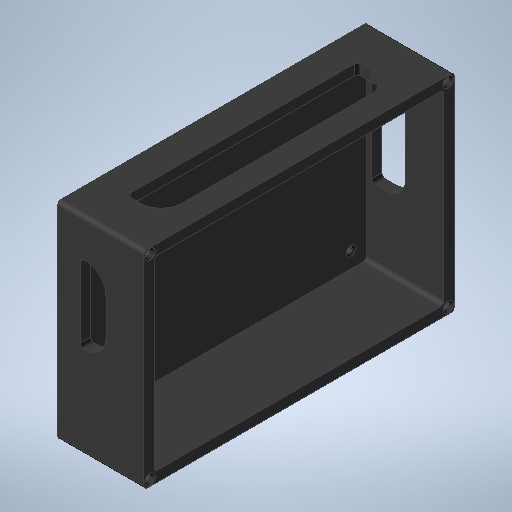
# Autodesk Inventor part: OCTOPUS_BOX
Saved by Autodesk Inventor 2025.2 (Build 292293000, 293)
## iProperties
Created: 2026-03-25
Part Number: OCTOPUS_BOX
Material: Generic
Document SubType Name: Modeling
Designer: composite
Density: 1 g/cm^3
Appearance: Default
Author: composite
Autodesk Inventor part; units mm, degrees
ref_plane "YZ Plane" through (0, 0, 0) normal (1, 0, 0) x (0, 1, 0)
ref_plane "XZ Plane" through (0, 0, 0) normal (0, 1, 0) x (-1, 0, 0)
ref_plane "XY Plane" through (0, 0, 0) normal (0, 0, 1) x (1, 0, 0)
sketch "Sketch1" plane through (0, 0, 0) normal (1, 0, 0) x (0, 1, 0)
  line L0 (0, 0) -> (120, 0)
  line L1 (120, 0) -> (120, -180)
  line L2 (120, -180) -> (0, -180)
  line L3 (0, -180) -> (0, 0)
  dimension "d0" = 120
  dimension "d1" = 180
  constraints: 8 end point, 2 parallel, 1 horizontal, 1 perpendicular
  measures "d0" distance of L1.end L2.end
  measures "d1" distance of L0.end L1.end
extrude "Extrusion1" add sketch "Sketch1" along normal blind 5
sketch "Sketch2" plane through (5, 0, 0) normal (1, 0, 0) x (0, 0, -1)
  line L0 (180, 0) -> (180, 120) projected
  line L1 (180, 120) -> (0, 120) projected
  line L2 (0, 120) -> (0, 0) projected
  line L3 (0, 0) -> (180, 0) projected
  line L4 (6, 114) -> (174, 114)
  line L5 (174, 114) -> (174, 6)
  line L6 (174, 6) -> (6, 6)
  line L7 (6, 6) -> (6, 114)
  dimension "d4" = 6
  constraints: 8 end point, 3 other
  measures "d4" distance between parallel lines of L1 L4
extrude "Extrusion2" add sketch "Sketch2" along normal blind 45
fillet "Fillet1" radius 2 8 edges at (27.5, 114, -174) (27.5, 114, -6) (27.5, 6, -6) (27.5, 6, -174) (25, 120, -180) (25, 120, 0) (25, 0, 0) (25, 0, -180)
sketch "Sketch3" plane through (5, 0, 0) normal (1, 0, 0) x (0, 0, -1)
  circle A0 centre (15, 105) radius 1.75
  arc A1 (172, 6) -> (174, 8) centre (172, 8) ccw projected
  line L0 (174, 8) -> (174, 112) projected
  arc A2 (174, 112) -> (172, 114) centre (172, 112) ccw projected
  line L1 (172, 114) -> (8, 114) projected
  arc A3 (8, 114) -> (6, 112) centre (8, 112) ccw projected
  line L2 (6, 112) -> (6, 8) projected
  arc A4 (6, 8) -> (8, 6) centre (8, 8) ccw projected
  line L3 (8, 6) -> (172, 6) projected
  circle A5 centre (165, 105) radius 1.75
  circle A6 centre (15, 15) radius 1.75
  circle A7 centre (165, 15) radius 1.75
  line L4 (15, 105) -> (15, 114) construction
  line L5 (15, 105) -> (6, 105) construction
  line L6 (165, 15) -> (165, 6) construction
  line L7 (165, 15) -> (174, 15) construction
  point P0 (0, 0)
  dimension "d8" = 3.5
  dimension "d12" = 150
  dimension "d15" = 90
  constraints: 8 end point, 4 centre point, 4 point on line, 3 perpendicular, 2 horizontal, 2 parallel, 2 vertical, 6 other
  measures "d8" diameter of A0
  measures "d12" distance of L4.start A5.centre
  measures "d15" distance of L4.start A6.centre
extrude "Extrusion3" cut sketch "Sketch3" against normal blind 20 contours A0 | A5 | A6 | A7
sketch "Sketch4" plane through (50, 0, 0) normal (1, 0, 0) x (0, 0, -1)
  arc A0 (178, 0) -> (180, 2) centre (178, 2) ccw projected
  line L0 (180, 2) -> (180, 118) projected
  arc A1 (180, 118) -> (178, 120) centre (178, 118) ccw projected
  line L1 (178, 120) -> (2, 120) projected
  arc A2 (2, 120) -> (0, 118) centre (2, 118) ccw projected
  line L2 (0, 118) -> (0, 2) projected
  arc A3 (0, 2) -> (2, 0) centre (2, 2) ccw projected
  line L3 (2, 0) -> (178, 0) projected
  line L4 (8, 114) -> (172, 114) projected
  arc A4 (174, 112) -> (172, 114) centre (172, 112) ccw projected
  line L5 (174, 112) -> (174, 8) projected
  arc A5 (172, 6) -> (174, 8) centre (172, 8) ccw projected
  line L6 (172, 6) -> (8, 6) projected
  arc A6 (6, 8) -> (8, 6) centre (8, 8) ccw projected
  line L7 (6, 8) -> (6, 112) projected
  arc A7 (8, 114) -> (6, 112) centre (8, 112) ccw projected
  circle A8 centre (3.5, 116.5) radius 2
  line L8 (8, 114) -> (172, 114) projected
  line L9 (6, 8) -> (6, 112) projected
  circle A9 centre (176.5, 116.5) radius 2
  circle A10 centre (176.5, 3.5) radius 2
  circle A11 centre (3.5, 3.5) radius 2
  point P0 (0, 0)
  dimension "d22" = 4
  dimension "d23" = 2.5
  dimension "d24" = 2.5
  dimension "d25" = 4
  dimension "d26" = 4
  dimension "d27" = 4
  dimension "d28" = 2.5
  dimension "d29" = 2.5
  dimension "d30" = 2.5
  dimension "d31" = 2.5
  dimension "d32" = 2.5
  dimension "d33" = 2.5
  constraints: 4 centre point
  measures "d22" diameter of A8
  measures "d23" distance from line of A8.centre L4
  measures "d24" distance from line of A8.centre L7
  measures "d25" diameter of A9
  measures "d26" diameter of A10
  measures "d27" diameter of A11
  measures "d28" distance from line of A11.centre L6
  measures "d29" distance from line of L7 A11.centre
  measures "d30" distance from line of L5 A10.centre
  measures "d31" distance from line of L6 A10.centre
  measures "d32" distance from line of A9.centre L5
  measures "d33" distance from line of L4 A9.centre
extrude "Extrusion4" cut sketch "Sketch4" against normal through all contours A8 | A9 | A10 | A11
chamfer "Chamfer1" distance 1 distance2 2 4 edges at (0, 116.5, -174.5) (0, 116.5, -1.5) (0, 3.5, -1.5) (0, 3.5, -174.5) measured on face at (0, 45.2711, -65.5165)
chamfer "Chamfer2" distance 1 distance2 2 4 edges at (50, 3.5, -174.5) (50, 3.5, -1.5) (50, 116.5, -1.5) (50, 116.5, -174.5) measured on face at (50, 3.4492, -117.3333)
chamfer "Chamfer3" distance 1 distance2 1 4 edges at (5, 105, -13.25) (5, 105, -163.25) (5, 15, -13.25) (5, 15, -163.25) measured on face at (5, 45.2711, -65.5165)
sketch "Sketch5" plane through (5, 114, -172) normal (0, -1, 0) x (1, 0, 0)
  line L0 (45, 170) -> (-5, 170) projected
  line L1 (45, -6) -> (45, 170) projected
  line L2 (-5, -6) -> (45, -6) projected
  line L3 (-5, -6) -> (-5, 170) projected
  line L4 (0, 164) -> (45, 164) projected
  line L5 (0, 0) -> (0, 164) projected
  line L6 (45, 0) -> (0, 0) projected
  line L7 (45, 164) -> (45, 0) projected
  line L8 (12, 149) -> (32, 149)
  line L9 (32, 149) -> (32, 15)
  line L10 (32, 15) -> (12, 15)
  line L11 (12, 15) -> (12, 149)
  point P0 (-5, 172)
  point P1 (22.5, 164)
  dimension "d45" = 15
  dimension "d46" = 15
  dimension "d47" = 12
  dimension "d48" = 20
  constraints: 8 end point, 2 parallel, 1 horizontal, 1 midpoint, 1 perpendicular
  measures "d45" distance between parallel lines of L6 L10
  measures "d46" distance from line of point (22.5, 164) L8
  measures "d47" distance between parallel lines of L5 L11
  measures "d48" distance between parallel lines of L11 L9
extrude "Extrusion5" cut sketch "Sketch5" against normal blind 45 contours L8 L9 L10 L11
sketch "Sketch6" plane through (5, 8, -174) normal (0, 0, 1) x (1, 0, 0)
  line L0 (-5, 95.25) -> (-5, 98.75) projected
  line L1 (-1, 98.75) -> (-1, 95.25) projected
  line L2 (45, 0) -> (0, 0) projected
  line L3 (45, 104) -> (45, 0) projected
  line L4 (0, 104) -> (45, 104) projected
  line L5 (0, 0) -> (0, 104) projected
  line L6 (3, 93.25) -> (23, 93.25)
  line L7 (23, 93.25) -> (23, 38.25)
  line L8 (23, 38.25) -> (3, 38.25)
  line L9 (3, 38.25) -> (3, 93.25)
  point P0 (-5, -8)
  dimension "d51" = 3
  dimension "d52" = 55
  dimension "d53" = 2
  dimension "d54" = 20
  constraints: 8 end point, 2 parallel, 1 horizontal, 1 perpendicular
  measures "d51" distance between parallel lines of L5 L9
  measures "d52" distance of L6.end L7.end
  measures "d53" distance from line of L1.end L6
  measures "d54" distance between parallel lines of L9 L7
extrude "Extrusion6" cut sketch "Sketch6" against normal through all contours L6 L7 L8 L9
sketch "Sketch7" plane through (5, 8, -6) normal (0, 0, -1) x (-1, 0, 0)
  line L0 (0, 0) -> (-45, 0) projected
  line L1 (0, 104) -> (0, 0) projected
  line L2 (-45, 104) -> (0, 104) projected
  line L3 (-45, 0) -> (-45, 104) projected
  line L4 (5, 98.75) -> (5, 95.25) projected
  line L5 (1, 95.25) -> (1, 98.75) projected
  line L6 (-8, 90.25) -> (-23, 90.25)
  line L7 (-23, 90.25) -> (-23, 45.25)
  line L8 (-23, 45.25) -> (-8, 45.25)
  line L9 (-8, 45.25) -> (-8, 90.25)
  point P0 (5, -8)
  dimension "d57" = 45
  dimension "d58" = 5
  dimension "d59" = 8
  dimension "d60" = 15
  constraints: 8 end point, 2 parallel, 1 horizontal, 1 perpendicular
  measures "d57" distance of L6.end L7.end
  measures "d58" distance from line of L5.start L6
  measures "d59" distance between parallel lines of L1 L9
  measures "d60" distance between parallel lines of L9 L7
extrude "Extrusion7" cut sketch "Sketch7" against normal blind 10 contours L9 L8 L7 L6
fillet "Fillet2" radius 12 6 edges at (37, 117, -23) (37, 117, -157) (28, 98.25, -3) (28, 53.25, -3) (28, 101.25, -177) (28, 46.25, -177)
fillet "Fillet3" radius 2 6 edges at (13, 98.25, -3) (17, 117, -157) (8, 101.25, -177) (8, 46.25, -177) (13, 53.25, -3) (17, 117, -23)
equation "\"d28\" = d23"
equation "\"d29\" = d28"
equation "\"d30\" = d29"
equation "\"d31\" = d29"
equation "\"d32\" = d23"
equation "\"d33\" = d23"
body "Solid1"
